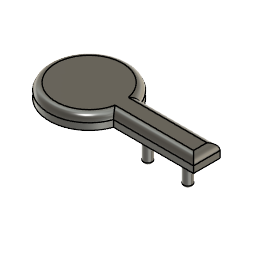
Power Button Cover (Autodesk Fusion 360 design; units mm, degrees)
part number: 2026-06-27-22-43-59-063
Autodesk Fusion 360 part; units mm, degrees
note: some values were not read from the file. Set by a fixed rule: which sketch regions a step uses.
sketch "Sketch1" plane through (0, 0, 0) normal (0, 0, 1) x (1, 0, 0)
  circle A0 centre (22, 0) radius 1.65
  circle A1 centre (37, 0) radius 1.65
  circle A2 centre (0, 0) radius 15
  line L0 (14.1421, 5) -> (44.1421, 5)
  line L1 (44.1421, 5) -> (44.1421, -5)
  line L2 (44.1421, -5) -> (14.1421, -5)
  line L3 (1.75, 0) -> (22.5, 0)
  dimension "d1" = 3.3
  dimension "d2" = 3.3
  dimension "d3" = 30
  dimension "d4" = 22
  dimension "d5" = 15
  dimension "d6" = 10
  dimension "d7" = 30
  constraint coincident A2.centre origin
  constraint horizontal L0
  constraint vertical L1
  constraint horizontal L2
  constraint coincident A2 L0.start
  constraint coincident A2 L2.end
  constraint equal L0 L2
  constraint coincident A0.centre L3
  constraint coincident A1.centre L3
  measures "d1" diameter of A1
  measures "d2" diameter of A0
  measures "d3" diameter of A2
  measures "d4" distance of A2.centre A0.centre
  measures "d5" distance of A0.centre A1.centre
  measures "d6" distance of L0.end L1.end
  measures "d7" distance of L1.end L2.end
extrude "Extrude1" add sketch "Sketch1" along normal blind 5 contours A0 | A1 | A2 | A2 L0 L1 L2
extrude "Extrude2" add sketch "Sketch1" against normal blind 10 contours A0 | A1
fillet "Fillet1" radius 2.5 4 edges at (-15, 0, 5) (29.1421, -5, 5) (29.1421, 5, 5) (44.1421, 0, 5)
fillet "Fillet2" radius 1 2 edges at (20.4617, 0.5967, -10) (35.4617, 0.5967, -10)
fillet "Fillet3" radius 0.5 2 edges at (20.4617, -0.5967, 0) (35.4617, -0.5967, 0)
